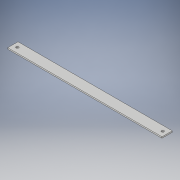
# Autodesk Inventor part: Long support flat
Saved by Autodesk Inventor 2017 (Build 210142000, 142)
## iProperties
Created: 2018-08-22
Part Number: Long support flat
Material: Generic
Document SubType Name: Modeling
Designer: sinner
Density: 1 g/cm^3
Appearance: Default
Author: sinner
Autodesk Inventor part; units mm, degrees
ref_plane "YZ Plane" through (0, 0, 0) normal (1, 0, 0) x (0, 1, 0)
ref_plane "XZ Plane" through (0, 0, 0) normal (0, 1, 0) x (-1, 0, 0)
ref_plane "XY Plane" through (0, 0, 0) normal (0, 0, 1) x (1, 0, 0)
sketch "Sketch1" plane through (0, 0, 0) normal (1, 0, 0) x (0, 1, 0)
  line L0 (0, 0) -> (3.2512, 0)
  line L1 (3.2512, 0) -> (3.2512, -25.4)
  line L2 (3.2512, -25.4) -> (0, -25.4)
  line L3 (0, -25.4) -> (0, 0)
  dimension "d0" = 3.2512
  dimension "d1" = 25.4
  constraints: 8 end point, 2 parallel, 1 horizontal, 1 perpendicular
  measures "d0" distance of L1.end L2.end
  measures "d1" distance of L0.end L1.end
extrude "Extrusion1" add sketch "Sketch1" along normal blind 381
sketch "Sketch2" plane through (0, 3.2512, 0) normal (0, 1, 0) x (1, 0, 0)
  line L0 (0, 25.4) -> (0, 0) projected
  line L1 (0, 12.7) -> (85.4474, 12.7) construction
  circle A0 centre (10.8949, 12.7) radius 3.175
  line L2 (0, 0) -> (381, 0) projected
  line L3 (190.5, 0) -> (190.5, 15.076) construction
  line L4 (381, 12.7) -> (295.5526, 12.7) construction
  circle A1 centre (370.1051, 12.7) radius 3.175
  dimension "d4" = 6.35
  dimension "d5" = 179.6051
  constraints: 6 end point, 3 symmetric about line, 2 centre point, 2 midpoint, 2 point on line, 1 horizontal, 1 vertical, 1 other
  measures "d4" diameter of A0
  measures "d5" distance from line of L3 A0.centre
extrude "Extrusion2" cut sketch "Sketch2" against normal blind 381
body "Solid1"
